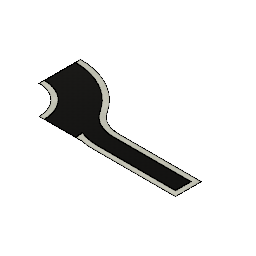
_On Ramp - Ruby.37fbb9db-0ea0-48d8-a00f-0c33148ef888 (Autodesk Fusion 360 design; units mm, degrees)
Autodesk Fusion 360 part; units mm, degrees
sketch "Sketch1" plane through (0, 0, 0) normal (0, 0, 1) x (1, 0, 0)
  circle A0 centre (0, 0) radius 660.4
  circle A1 centre (0, 0) radius 1270
  line L0 (0, 0) -> (0, 1270)
  line L1 (0, 0) -> (1270, 0)
  circle A2 centre (1624.8851, 1042.2056) radius 660.4
  circle A3 centre (1624.8851, 1042.2056) radius 965.2
  line L2 (1624.8851, 1042.2056) -> (1624.8851, 77.0056)
  line L3 (1624.8851, 77.0056) -> (3148.8851, 77.0056)
  line L4 (3148.8851, 77.0056) -> (3148.8851, 381.8056)
  line L5 (3148.8851, 381.8056) -> (1624.8851, 381.8056)
  line L6 (1624.8851, 381.8056) -> (1624.8851, 77.0056)
  dimension "d1" = 1320.8
  dimension "d2" = 609.6
  dimension "d3" = 1320.8
  dimension "d4" = 304.8
  dimension "d5" = 1524
  dimension "d6" = 304.8
  constraint coincident A0.centre A1.centre
  constraint coincident A1 L0.end
  constraint vertical L0
  constraint coincident A1 L1.end
  constraint perpendicular L0 L1
  constraint tangent A1 A2
  constraint coincident A2.centre A3.centre
  constraint coincident A3 L2.end
  constraint vertical L2
  constraint horizontal L3
  constraint vertical L4
  constraint horizontal L5
  constraint vertical L6
  measures "d1" diameter of A0
  measures "d3" diameter of A2
  measures "d5" distance of L2.end L3.end
  measures "d6" distance of L2.end L5.end
extrude "Extrude1" add sketch "Sketch1" along normal blind 6.096 contours A0 A1 L0 L1 A3 | A1 A3 | A1 A2 A3 L2 L6 | A3 L2 L5 L6 | A3 L3 L4 L5 makes body 1
sketch "Sketch2" plane through (0, 0, 6.096) normal (0, 0, 1) x (-1, 0, 0)
  line L0 (-660.4, 0) -> (-1270, 0)
  arc A0 (-1270, 0) -> (-1261.3364, -148.0897) centre (0, 0) ccw
  arc A1 (-1261.3364, -148.0897) -> (-1624.8851, -77.0056) centre (-1624.8851, -1042.2056) ccw
  line L1 (-1624.8851, -77.0056) -> (-3148.8851, -77.0056)
  line L2 (-3148.8851, -77.0056) -> (-3148.8851, -381.8056)
  line L3 (-3148.8851, -381.8056) -> (-1624.8851, -381.8056)
  arc A2 (-1069.0034, -685.6616) -> (-1624.8851, -381.8056) centre (-1624.8851, -1042.2056) ccw
  arc A3 (-1069.0034, -685.6616) -> (0, -1270) centre (0, 0) ccw
  line L4 (0, -1270) -> (0, -660.4)
  arc A4 (-660.4, 0) -> (0, -660.4) centre (0, 0) ccw
  arc A5 (-549.486, 101.6) -> (101.6, -549.486) centre (0, 0) ccw
  line L5 (101.6, -1367.8319) -> (101.6, -549.486)
  arc A6 (-1154.5236, -740.5145) -> (101.6, -1367.8319) centre (0, 0) ccw
  arc A7 (-1154.5236, -740.5145) -> (-1624.8851, -483.4056) centre (-1624.8851, -1042.2056) ccw
  line L6 (-3250.4851, -483.4056) -> (-1624.8851, -483.4056)
  line L7 (-3250.4851, 24.5944) -> (-3250.4851, -483.4056)
  line L8 (-1624.8851, 24.5944) -> (-3250.4851, 24.5944)
  arc A8 (-1371.5873, -5.913) -> (-1624.8851, 24.5944) centre (-1624.8851, -1042.2056) ccw
  arc A9 (-1367.8319, 101.6) -> (-1371.5873, -5.913) centre (0, 0) ccw
  line L9 (-549.486, 101.6) -> (-1367.8319, 101.6)
  line L10 (-549.486, 101.6) -> (-1383.9809, 101.6)
  line L11 (-1383.9809, 101.6) -> (-1383.9809, 0)
  line L12 (-1383.9809, 0) -> (-549.486, 0)
  line L13 (-549.486, 0) -> (-549.486, 101.6)
  line L14 (101.6, -549.486) -> (0, -549.486)
  line L15 (0, -549.486) -> (0, -1422.4)
  line L16 (0, -1422.4) -> (101.6, -1422.4)
  line L17 (101.6, -1422.4) -> (101.6, -549.486)
  dimension "d9" = 101.6
  dimension "d10" = 101.6
  constraint horizontal L10
  constraint vertical L11
  constraint horizontal L12
  constraint vertical L13
  constraint horizontal L14
  constraint vertical L15
  constraint horizontal L16
  constraint vertical L17
  measures "d10" distance of A5.start L12.end
extrude "Extrude1'" add sketch "Sketch2" against normal blind 6.35 separate body contours A4 A5 L12 L15 | A0 A1 L1 L2 L3 A2 A3 A6 A7 L6 L7 L8 A8 A9 L12 L15 makes body 2 at (2674.7518, 9.2723, 6.096) makes body 3 at (31.3282, 624.2927, 6.096) in component "On Ramp"
copy_body "CutPasteBodies1" bodies 1 removing the originals makes body 4 in component "On Ramp"
component "On Ramp" placed x (1, 0, 0) y (0, 1, 0) z (0, 0, 1) at (0, 0, 0)
